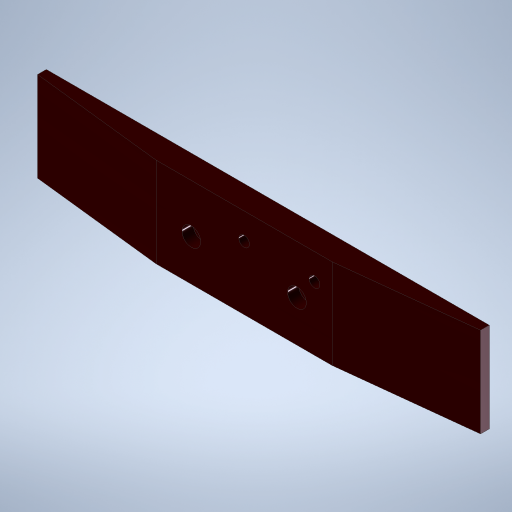
# Autodesk Inventor part: ZED_mount_V2
Saved by Autodesk Inventor 2024 (Build 280153000, 153)
## iProperties
Created: 2024-03-08
Part Number: ZED_mount_V2
Material: Generic
Document SubType Name: Modeling
Designer: critt
Density: 1 g/cm^3
Appearance: Default
Author: critt
## iProperties of the stored document ZED_mount_V2_3DPrint.ipt
Created: 2024-03-08
Part Number: ZED_mount_V2_3DPrint
Material: Generic
Document SubType Name: Modeling
Designer: critt
Density: 1 g/cm^3
Appearance: Default
Author: critt
Autodesk Inventor part; units mm, degrees
ref_plane "YZ Plane" through (0, 0, 0) normal (1, 0, 0) x (0, 1, 0)
ref_plane "XZ Plane" through (0, 0, 0) normal (0, 1, 0) x (-1, 0, 0)
sketch "Sketch1" plane through (0, 0, 0) normal (0, 0, 1) x (1, 0, 0)
  line L0 (0, 0) -> (151, 0)
  line L1 (151, 0) -> (151, 30.623)
  line L2 (151, 30.623) -> (0, 30.623)
  line L3 (0, 30.623) -> (0, 0)
  dimension "d0" = 151
  dimension "d1" = 30.623
  constraints: 8 end point, 2 parallel, 1 horizontal, 1 perpendicular
  measures "d0" distance between parallel lines of L3 L1
  measures "d1" distance between parallel lines of L0 L2
extrude "Extrusion1" add sketch "Sketch1" along normal blind 3
ref_plane "Work Plane2" through (0, 0, 8.08) normal (0, 0, 1) x (1, 0, 0)
sketch "Sketch2" plane through (0, 0, 8.08) normal (0, 0, 1) x (1, 0, 0)
  line L0 (151, 0) -> (151, 30.623) construction
  line L1 (151, 30.623) -> (0, 30.623) construction
  line L2 (0, 30.623) -> (0, 0) projected
  line L3 (0, 0) -> (151, 0) construction
  line L4 (45.5, 30.623) -> (105.5, 30.623)
  line L5 (105.5, 30.623) -> (105.5, 0)
  line L6 (105.5, 0) -> (45.5, 0)
  line L7 (45.5, 0) -> (45.5, 30.623)
  line L8 (45.5, 15.3115) -> (0, 15.3115) construction
  line L9 (105.5, 15.3115) -> (151, 15.3115) construction
  dimension "d6" = 60
  constraints: 12 end point, 4 midpoint, 2 parallel, 2 point on line, 1 collinear, 1 horizontal, 1 perpendicular
  measures "d6" distance of L9.start L8.start
loft "Loft1" add profiles "Sketch2" section 1 edges at (151, 15.3115, 3) (75.5, 30.623, 3) (0, 15.3115, 3) (75.5, 0, 3)
sketch "Sketch7" plane through (0, 0, 0) normal (0, 0, -1) x (-1, 0, 0)
  circle A0 centre (-93.5, 14.08) radius 1.8
  circle A1 centre (-57.5, 14.08) radius 1.8
  line L0 (0, 0) -> (-151, 0) projected
  line L1 (-151, 0) -> (-151, 30.623) projected
  line L2 (0, 30.623) -> (0, 0) projected
  dimension "d25" = 14.08
  dimension "d26" = 14.08
  dimension "d27" = 57.5
  dimension "d28" = 3.6
  dimension "d29" = 57.5
  dimension "d30" = 3.6
  constraints: 2 centre point
  measures "d25" distance from line of L0 A0.centre
  measures "d26" distance from line of A1.centre L0
  measures "d27" distance from line of L1 A0.centre
  measures "d28" diameter of A0
  measures "d29" distance from line of L2 A1.centre
  measures "d30" diameter of A1
extrude "Extrusion4" cut sketch "Sketch7" along normal mid plane 225.25
sketch "Sketch8" plane through (45.5, 30.623, 8.08) normal (0, 0, 1) x (1, 0, 0)
  circle A0 centre (48, -16.543) radius 1.8 projected
  circle A1 centre (12, -16.543) radius 1.8 projected
  line L0 (60, 0) -> (60, -30.623) projected
  line L1 (0, 0) -> (60, 0) projected
  line L2 (0, -30.623) -> (0, 0) projected
  line L3 (60, -30.623) -> (0, -30.623) projected
  circle A2 centre (12, -16.543) radius 3.175
  circle A3 centre (48, -16.543) radius 3.175
  point P0 (-45.5, -30.623)
  dimension "d33" = 6.35
  dimension "d34" = 6.35
  constraints: 2 centre point, 2 coincident
  measures "d33" diameter of A2
  measures "d34" diameter of A3
extrude "Extrusion5" cut sketch "Sketch8" against normal blind 3.81 contours A0 | A1 | A2 | A3
sketch "Sketch9" plane through (0, 0, 0) normal (0, 0, -1) x (-1, 0, 0)
  circle A0 centre (-75.5, 21.7) radius 1.8
  circle A1 centre (-99.5, 21.7) radius 1.8
  circle A2 centre (-93.5, 14.08) radius 1.8 projected
  circle A3 centre (-57.5, 14.08) radius 1.8 projected
  line L0 (-151, 0) -> (-151, 30.623) projected
  line L1 (0, 0) -> (-151, 0) projected
  line L2 (0, 30.623) -> (0, 0) projected
  line L3 (-151, 30.623) -> (0, 30.623) projected
  line L4 (-75.5, 21.7) -> (-75.5, 0) construction
  line L5 (-75.5, 21.7) -> (-99.5, 21.7) construction
  dimension "d37" = 3.6
  dimension "d38" = 3.6
  dimension "d40" = 24
  dimension "d43" = 7.62
  constraints: 4 end point, 2 centre point, 1 horizontal, 1 midpoint, 1 vertical
  measures "d37" diameter of A0
  measures "d38" diameter of A1
  measures "d40" distance of L4.start L5.end
  measures "d43" distance from line of A2.centre L5
extrude "Extrusion6" cut sketch "Sketch9" along normal mid plane 73.66 contours A0 | A1
sketch "Sketch11" plane through (0, 0, 0) normal (0, 0, -1) x (-1, 0, 0)
  circle A0 centre (-99.5, 21.7) radius 1.8 projected
  circle A1 centre (-75.5, 21.7) radius 1.8 projected
  circle A2 centre (-93.5, 14.08) radius 1.8 projected
  circle A3 centre (-57.5, 14.08) radius 1.8 projected
  line L0 (-151, 0) -> (-151, 30.623) projected
  line L1 (0, 0) -> (-151, 0) projected
  line L2 (0, 30.623) -> (0, 0) projected
  line L3 (-151, 30.623) -> (0, 30.623) projected
  circle A4 centre (-75.5, 21.7) radius 3.175
  circle A5 centre (-99.5, 21.7) radius 3.175
  dimension "d44" = 6.35
  dimension "d45" = 6.35
  constraints: 2 centre point, 2 coincident
  measures "d44" diameter of A4
  measures "d45" diameter of A5
extrude "Extrusion7" cut sketch "Sketch11" against normal blind 3.81 contours A0 | A1 | A4 | A5
body "Solid1"
